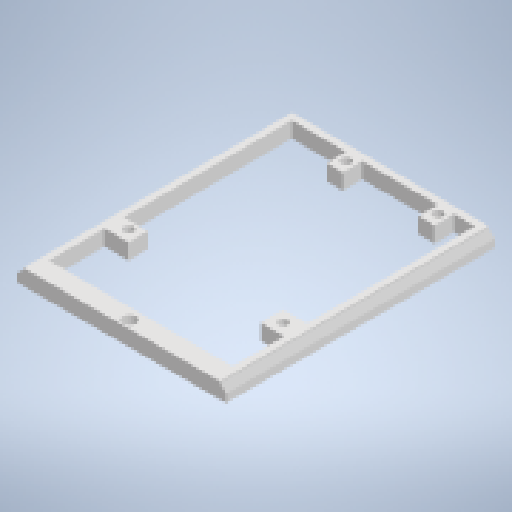
# Autodesk Inventor part: tampa
Saved by Autodesk Inventor 2025.1 (Build 291241000, 241)
## iProperties
Created: 2024-03-03
Part Number: tampa
Material: Genérico
Document SubType Name: Modeling
Designer: joaov
Density: 1 g/cm^3
Appearance: Padrão
Author: joaov
Autodesk Inventor part; units mm, degrees
ref_plane "YZ Plane" through (0, 0, 0) normal (1, 0, 0) x (0, 1, 0)
ref_plane "XZ Plane" through (0, 0, 0) normal (0, 1, 0) x (-1, 0, 0)
ref_plane "XY Plane" through (0, 0, 0) normal (0, 0, 1) x (1, 0, 0)
sketch "Esboço1" plane through (0, 0, 0) normal (0, 0, 1) x (1, 0, 0)
  line L0 (2.9, 0) -> (65.7, 0)
  line L1 (2.9, 0) -> (2.7, 0)
  line L2 (65.7, 0) -> (65.9, 0)
  line L3 (4.6, 4.8) -> (64, 4.8)
  line L4 (64, 4.8) -> (64.2, 4.8)
  line L5 (65.9, 0) -> (66.1, 0)
  line L6 (66.1, 0) -> (66.1, 2.4)
  line L7 (66.1, 2.4) -> (64.2, 4.3)
  line L8 (64.2, 4.8) -> (64.2, 4.3)
  line L9 (2.9, 0) -> (2.7, 0)
  line L10 (4.6, 4.8) -> (4.4, 4.8)
  line L11 (2.7, 0) -> (2.5, 0)
  line L12 (2.5, 0) -> (2.5, 2.4)
  line L13 (2.5, 2.4) -> (4.4, 4.3)
  line L14 (4.4, 4.8) -> (4.4, 4.3)
  point P0 (61.9143, 91.5369)
  constraints: 30 end point, 4 horizontal, 1 perpendicular
extrude "Extrusão1" add sketch "Esboço1" along normal blind 96.6
sketch "Esboço3" plane through (4.4, 4.8, 0) normal (0, 1, 0) x (1, 0, 0)
  line L0 (64.2, -96.6) -> (-4.4, -96.6)
  line L1 (-1.9, -96.6) -> (61.7, -96.6)
  line L2 (29.9, -96.6) -> (29.9, -94.2)
  circle A0 centre (51.4, -94.2) radius 1.45
  line L3 (29.9, -96.6) -> (29.9, -91.8)
  line L4 (29.9, -94.2) -> (51.4, -94.2)
  line L5 (29.9, -94.2) -> (8.4, -94.2)
  circle A1 centre (8.4, -94.2) radius 1.45
  line L6 (0.4, -91.8) -> (59.4, -91.8)
  line L7 (61.7, -96.6) -> (-1.9, -96.6)
  circle A2 centre (29.9, -94.2) radius 1.45
  point P0 (-1.9, 0)
  point P1 (61.7, 0)
  dimension "d104" = 2.4
  dimension "d105" = 2.4
  dimension "d140" = 2.9
  constraints: 16 end point, 3 centre point, 3 coincident
  measures "d104" distance between parallel lines of L0 L5
  measures "d105" distance between parallel lines of L4 L6
  measures "d140" diameter of A2
extrude "Extrusão3" cut sketch "Esboço3" against normal through all contours A2 L5 L2 | L2 L4 A2 | L5 A2 L3 | L3 A2 L4
sketch "Esboço4" plane through (4.4, 4.8, 0) normal (0, 1, 0) x (1, 0, 0)
  line L0 (-1.9, 0) -> (61.7, 0) projected
  line L1 (29.9, 0) -> (29.9, -4.8)
  line L2 (29.9, -4.8) -> (29.9, -14.8)
  line L3 (29.9, -14.8) -> (4.9, -14.8)
  line L4 (29.9, -14.8) -> (54.9, -14.8)
  line L5 (4.9, -14.8) -> (4.9, -4.8)
  line L6 (4.9, -4.8) -> (29.9, -4.8)
  line L7 (29.9, -4.8) -> (54.9, -4.8)
  line L8 (54.9, -4.8) -> (54.9, -14.8)
  line L9 (61.7, 0) -> (61.7, -96.6) projected
  line L10 (61.7, -14.8) -> (-1.9, -14.8)
  line L11 (-1.9, -14.8) -> (-1.9, 0)
  line L12 (-1.9, 0) -> (61.7, 0)
  line L13 (61.7, 0) -> (61.7, -14.8)
  point P0 (-4.4, 0)
  dimension "d51" = 4.8
  dimension "d52" = 10
  dimension "d53" = 25
  dimension "d54" = 25
  constraints: 24 end point, 4 perpendicular, 3 point on line, 2 horizontal, 2 parallel, 2 vertical, 1 midpoint
  measures "d51" distance of L1.start L1.end
  measures "d52" distance of L1.end L2.end
  measures "d53" distance of L2.end L3.end
  measures "d54" distance of L2.end L4.end
extrude "Extrusão4" cut sketch "Esboço4" against normal through all
sketch "Esboço5" plane through (4.4, 4.8, 0) normal (0, 1, 0) x (1, 0, 0)
  line L0 (59.8, 0) -> (59.8, -96.6) projected
  line L1 (0, 0) -> (0, -96.6) projected
  line L2 (-1.9, -96.6) -> (61.7, -96.6) projected
  line L3 (-1.9, 0) -> (61.7, 0) projected
  line L4 (29.9, -85.38) -> (3.23, -85.38)
  line L5 (29.9, -85.38) -> (56.57, -85.38)
  line L6 (3.23, -85.38) -> (3.23, -70.14)
  line L7 (3.23, -70.14) -> (4.23, -70.14)
  line L8 (4.23, -70.14) -> (5.83, -70.14)
  line L9 (56.57, -85.38) -> (56.57, -16.8)
  line L10 (3.23, -70.14) -> (3.23, -16.8)
  line L11 (3.23, -16.8) -> (21.01, -16.8)
  line L12 (3.23, -16.8) -> (48.95, -16.8)
  line L13 (21.01, -16.8) -> (21.01, -17.8)
  line L14 (48.95, -16.8) -> (48.95, -17.8)
  line L15 (21.01, -17.8) -> (21.01, -19.4)
  line L16 (48.95, -17.8) -> (48.95, -19.4)
  circle A0 centre (21.01, -19.4) radius 1.45
  circle A1 centre (48.95, -19.4) radius 1.45
  line L17 (5.83, -70.14) -> (5.83, -70.44)
  circle A2 centre (5.83, -70.44) radius 1.45
  line L18 (53.97, -70.14) -> (53.97, -71.54)
  circle A3 centre (53.97, -71.54) radius 1.45
  line L19 (4.9, -14.8) -> (54.9, -14.8) projected
  point P0 (-4.4, 0)
  dimension "d60" = 53.34
  dimension "d61" = 15.24
  dimension "d62" = 1
  dimension "d63" = 1.6
  dimension "d64" = 68.58
  dimension "d65" = 17.78
  dimension "d67" = 45.72
  dimension "d69" = 1
  dimension "d70" = 1
  dimension "d71" = 1.6
  dimension "d72" = 1.6
  dimension "d73" = 2.9
  dimension "d74" = 2.9
  dimension "d77" = 68.58
  dimension "d86" = 0.3
  dimension "d87" = 2.9
  dimension "d88" = 1.4
  dimension "d89" = 2.9
  constraints: 30 end point, 6 vertical, 5 coincident, 4 centre point, 4 perpendicular, 2 horizontal, 1 parallel
  measures "d60" distance of L5.end L4.end
  measures "d61" distance of L4.end L6.end
  measures "d62" distance of L6.end L7.end
  measures "d63" distance of L7.end L8.end
  measures "d64" distance of L5.end L9.end
  measures "d65" distance of L10.end L11.end
  measures "d67" distance of L10.end L12.end
  measures "d69" distance of L11.end L13.end
  measures "d70" distance of L12.end L14.end
  measures "d71" distance of L13.end L15.end
  measures "d72" distance of L14.end L16.end
  measures "d73" diameter of A0
  measures "d74" diameter of A1
  measures "d77" distance of L10.end L4.end
  measures "d86" distance of L17.start L17.end
  measures "d87" diameter of A2
  measures "d88" distance of L18.start L18.end
  measures "d89" diameter of A3
extrude "Extrusão5" cut sketch "Esboço5" against normal through all contours A2 | A1 | A0 | A3
sketch "Esboço10" plane through (4.4, 4.8, 96.6) normal (0, 1, 0) x (1, 0, 0)
  circle A0 centre (53.97, 25.06) radius 1.45 projected
  circle A1 centre (5.83, 26.16) radius 1.45 projected
  circle A2 centre (48.95, 77.2) radius 1.45 projected
  line L0 (48.95, 77.2) -> (48.95, 75.75)
  line L1 (48.95, 75.75) -> (48.95, 73.75)
  circle A3 centre (21.01, 77.2) radius 1.45 projected
  line L2 (21.01, 75.75) -> (21.01, 73.75)
  line L3 (59.8, 81.8) -> (59.8, 0) projected
  line L4 (59.8, 40.9) -> (57.8, 40.9)
  line L5 (0, 81.8) -> (0, 0) projected
  line L6 (0, 40.9) -> (2, 40.9)
  line L7 (51.4, 3.85) -> (51.4, 5.85)
  line L8 (57.8, 40.9) -> (57.8, 73.75)
  line L9 (57.8, 73.75) -> (48.95, 73.75)
  line L10 (48.95, 73.75) -> (21.01, 73.75)
  line L11 (21.01, 73.75) -> (2, 73.75)
  line L12 (2, 73.75) -> (2, 40.9)
  line L13 (53.97, 28.51) -> (50.52, 28.51)
  line L14 (50.52, 28.51) -> (50.52, 25.06)
  line L15 (51.4, 5.85) -> (57.8, 5.85)
  line L16 (57.8, 40.9) -> (57.8, 28.51)
  line L17 (57.8, 28.51) -> (53.97, 28.51)
  line L18 (57.8, 5.85) -> (57.8, 21.61)
  line L19 (57.8, 21.61) -> (53.97, 21.61)
  line L20 (53.97, 21.61) -> (50.52, 21.61)
  line L21 (50.52, 21.61) -> (50.52, 25.06)
  line L22 (2, 40.9) -> (2, 29.61)
  line L23 (2, 22.71) -> (2, 5.85)
  line L24 (2, 5.85) -> (51.4, 5.85)
  line L25 (2, 29.61) -> (5.83, 29.61)
  line L26 (9.28, 29.61) -> (9.28, 26.16)
  line L27 (9.28, 22.71) -> (5.83, 22.71)
  line L28 (5.83, 22.71) -> (2, 22.71)
  line L29 (9.28, 22.71) -> (9.28, 26.16)
  line L30 (9.28, 29.61) -> (5.83, 29.61)
  line L31 (57.8, 21.61) -> (57.8, 28.51)
  point P0 (-4.4, 96.6)
  dimension "d108" = 2
  dimension "d109" = 2
  dimension "d110" = 2
  dimension "d111" = 2
  constraints: 60 end point, 11 perpendicular, 8 vertical, 6 horizontal, 4 point on line, 2 collinear, 2 midpoint, 2 vertical alignment, 1 parallel, 2 other
  measures "d108" distance of L0.end L1.end
  measures "d109" distance of L2.start L2.end
  measures "d110" distance of L4.start L4.end
  measures "d111" distance of L6.start L6.end
extrude "Extrusão10" cut sketch "Esboço10" against normal through all contours L9 L8 L16 L17 L13 L14 L21 L20 L19 L18 L15 L24 L23 L28 L27 L29 L26 L30 L25 L22 L12 L11 L10
sketch "Esboço13" plane through (4.4, 4.8, 96.6) normal (0, 1, 0) x (1, 0, 0)
  circle A0 centre (48.95, 77.2) radius 1.45 projected
  line L0 (51.4, 77.2) -> (51.4, 73.75)
  line L1 (51.4, 79.65) -> (51.4, 77.2)
  line L2 (57.8, 77.2) -> (57.8, 79.65)
  line L3 (57.8, 79.65) -> (51.4, 79.65)
  circle A1 centre (21.01, 77.2) radius 1.45 projected
  line L4 (23.46, 77.2) -> (23.46, 73.75)
  line L5 (23.46, 77.2) -> (23.46, 79.65)
  line L6 (46.5, 77.2) -> (46.5, 73.75)
  line L7 (46.5, 77.2) -> (46.5, 79.65)
  line L8 (46.5, 79.65) -> (23.46, 79.65)
  line L9 (17.9739, 79.65) -> (2, 79.65)
  line L10 (2, 73.75) -> (2, 29.61) projected
  line L11 (2, 79.65) -> (2, 73.75)
  line L12 (2, 73.75) -> (17.9739, 73.75)
  line L13 (18.56, 77.2) -> (18.56, 73.75)
  line L14 (18.56, 73.75) -> (17.9739, 73.75)
  line L15 (18.56, 77.2) -> (18.56, 79.65)
  line L16 (18.56, 79.65) -> (17.9739, 79.65)
  line L17 (9.28, 22.71) -> (9.28, 29.61) projected
  line L18 (9.28, 29.61) -> (9.28, 28.61)
  line L19 (9.28, 28.61) -> (2, 28.61)
  line L20 (2, 28.61) -> (2, 29.61)
  line L21 (9.28, 29.61) -> (2, 29.61)
  line L22 (57.8, 28.51) -> (57.8, 73.75) projected
  line L23 (57.8, 77.2) -> (57.8, 73.75)
  line L24 (57.8, 73.75) -> (51.4, 73.75)
  line L25 (2, 73.75) -> (57.8, 73.75) projected
  line L26 (51.4, 73.75) -> (2, 73.75)
  point P0 (-4.4, 96.6)
  dimension "d139" = 1
  constraints: 46 end point, 8 vertical, 7 perpendicular, 3 collinear, 2 point on line, 1 horizontal
  measures "d139" distance of L17.end L18.end
extrude "Extrusão12" cut sketch "Esboço13" against normal through all contours L1 L3 L2 L23 L24 L0 | L21 L17 L19 L20 | L14 L12 L11 L9 L16 L15 L13 | L25 L4 L5 L8 L7 L6
sketch "Esboço15" plane through (4.4, 4.8, 96.6) normal (0, 1, 0) x (1, 0, 0)
  circle A0 centre (29.9, 2.4) radius 1.45 projected
  circle A1 centre (29.9, 2.4) radius 1.45
  circle A2 centre (29.9, 2.4) radius 1.95
  point P0 (-4.4, 96.6)
  dimension "d142" = 3.9
  constraints: 2 centre point, 2 coincident
  measures "d142" diameter of A2
extrude "Extrusão13" cut sketch "Esboço15" against normal blind 3
